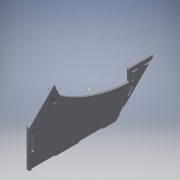
# Autodesk Inventor part: lateral
Saved by Autodesk Inventor 2016 (Build 200138000, 138)
## iProperties
Created: 2017-06-05
Part Number: lateral
Material: Genérico
Document SubType Name: Modeling
Designer: Fabio
Density: 1 g/cm^3
Appearance: Padrão
Author: Fabio
Autodesk Inventor part; units mm, degrees
ref_plane "YZ Plane" through (0, 0, 0) normal (1, 0, 0) x (0, 1, 0)
ref_plane "XZ Plane" through (0, 0, 0) normal (0, 1, 0) x (-1, 0, 0)
ref_plane "XY Plane" through (0, 0, 0) normal (0, 0, 1) x (1, 0, 0)
sketch "Esboço1" plane through (0, 0, 0) normal (1, 0, 0) x (0, 1, 0)
  line L0 (-220, 137.5) -> (220, 137.5)
  line L1 (220, 137.5) -> (220, -137.5)
  line L2 (220, -137.5) -> (-220, -137.5)
  line L3 (-220, -137.5) -> (-220, 137.5)
  point P0 (0, 0)
  point P1 (220, 0)
  point P2 (0, -137.5)
  dimension "d0" = 440
  dimension "d1" = 275
  constraints: 8 end point, 2 midpoint, 2 parallel, 1 horizontal, 1 horizontal alignment, 1 perpendicular, 1 vertical alignment
  measures "d0" distance between parallel lines of L3 L1
  measures "d1" distance between parallel lines of L0 L2
extrude "Extrusão1" add sketch "Esboço1" along normal blind 8
sketch "Esboço2" plane through (8, 0, 0) normal (1, 0, 0) x (0, 0, -1)
  line L0 (124.1566, 220.0243) -> (0, 220)
  line L1 (137.5, 220) -> (-137.5, 220) projected
  line L2 (0, 135) -> (42.099, 135)
  line L3 (0, 135) -> (0, 220)
  line L4 (-137.5, -220) -> (137.5, -220) projected
  line L5 (137.5, 220) -> (137.5, -220)
  line L6 (137.5, -220) -> (-137.5, -220)
  line L7 (-137.5, -220) -> (-137.5, -140)
  line L8 (-137.5, 220) -> (-137.5, -220) projected
  arc A0 (-137.5, -140) -> (-37.6456, -108.3893) centre (-153.3983, 83.74) ccw
  arc A1 (-37.6456, -108.3893) -> (42.099, 135) centre (-427.017, 153.9438) ccw
  line L9 (137.5, -220) -> (137.5, 220) projected
  line L10 (137.5, -120) -> (-12.5, -120)
  line L11 (-12.5, -120) -> (-127.5, -163)
  line L12 (-127.5, -163) -> (-127.5, -210)
  line L13 (-127.5, -210) -> (137.5, -210)
  line L14 (10, 145) -> (50.5, 145)
  line L15 (50.5, 145) -> (137.5, 98)
  line L16 (137.5, 98) -> (137.5, 210)
  line L17 (10, 210) -> (10, 145)
  line L18 (10, 210) -> (137.5, 210)
  line L19 (137.5, 98) -> (137.5, 210)
  point P0 (0, 0)
  dimension "d8" = 137.5
  dimension "d9" = 275
  dimension "d10" = 80
  dimension "d11" = 85
  dimension "d12" = 10
  dimension "d13" = 10
  dimension "d14" = 10
  dimension "d15" = 65
  dimension "d16" = 150
  dimension "d17" = 10
  dimension "d18" = 10
  dimension "d19" = 90
  dimension "d20" = 115
  dimension "d21" = 47
  dimension "d22" = 112
  dimension "d23" = 87
  dimension "d24" = 420
  dimension "d25" = 40.5
  constraints: 32 end point, 5 point on line, 4 perpendicular, 4 point on circle, 2 centre point, 2 collinear, 2 horizontal, 2 vertical, 1 midpoint, 1 parallel
  measures "d8" distance between parallel lines of L5 L3
  measures "d9" distance between parallel lines of L5 L7
  measures "d10" distance of L4.start L7.end
  measures "d11" distance between parallel lines of L1 L2
  measures "d12" distance between parallel lines of L2 L14
  measures "d13" distance between parallel lines of L1 L18
  measures "d14" distance between parallel lines of L3 L17
  measures "d15" distance between parallel lines of L18 L14
  measures "d16" distance of L10.start L10.end
  measures "d17" distance between parallel lines of L8 L12
  measures "d18" distance between parallel lines of L4 L13
  measures "d19" distance between parallel lines of L13 L10
  measures "d20" horizontal distance of L10.end L11.end
  measures "d21" distance from line of L11.end L13
  measures "d22" distance of L16.end L15.end
  measures "d23" horizontal distance of L14.end L15.end
  measures "d24" distance between parallel lines of L13 L18
  measures "d25" distance of L14.start L14.end
extrude "Extrusão2" cut sketch "Esboço2" against normal blind 10 contours L3 L2 A1 A0 L8 L1
fillet "Arredondamento1" radius 4 7 edges at (4, 135, 0) (4, 135, -42.099) (4, 220, 0) (4, 220, -137.5) (4, -140, 137.5) (4, -220, 137.5) (4, -220, -137.5)
fillet "Arredondamento2" radius 40 1 edges at (4, -108.3893, 37.6456)
sketch "Esboço3" plane through (0, 0, 0) normal (-1, 0, 0) x (0, 0, 1)
  point P0 (0, 0)
sketch "Esboço4" plane through (0, 0, 0) normal (-1, 0, 0) x (0, 0, 1)
  point P0 (0, 0)
sketch "Esboço5" plane through (8, 0, 0) normal (1, 0, 0) x (0, 0, -1)
  line L0 (-123.5, -210) -> (-119.5, -210)
  line L1 (-119.5, -210) -> (-119.5, -194)
  line L2 (-119.5, -194) -> (-123.5, -194)
  line L3 (-123.5, -194) -> (-123.5, -210)
  line L4 (-137.5, -143.6953) -> (-137.5, -216) projected
  line L5 (-133.5, -220) -> (133.5, -220) projected
  circle A0 centre (-123.5, -194) radius 1
  circle A1 centre (-119.5, -194) radius 1
  circle A2 centre (-123.5, -210) radius 1
  circle A3 centre (-119.5, -210) radius 1
  line L6 (-123.5, -178) -> (-119.5, -178)
  line L7 (-119.5, -178) -> (-119.5, -162)
  line L8 (-119.5, -162) -> (-123.5, -162)
  line L9 (-123.5, -162) -> (-123.5, -178)
  circle A4 centre (-119.5, -178) radius 1
  circle A5 centre (-123.9206, -178) radius 1
  circle A6 centre (-123.5, -162) radius 1
  circle A7 centre (-119.5, -162) radius 1
  point P0 (0, 0)
  dimension "d26" = 14
  dimension "d27" = 10
  dimension "d28" = 4
  dimension "d29" = 16
  dimension "d30" = 2
  dimension "d31" = 2
  dimension "d32" = 2
  dimension "d33" = 2
  dimension "d36" = 4
  dimension "d37" = 16
  dimension "d38" = 16
  dimension "d39" = 2
  dimension "d40" = 2
  dimension "d41" = 2
  dimension "d42" = 2
  constraints: 16 end point, 8 centre point, 7 coincident, 4 parallel, 2 horizontal, 2 perpendicular, 1 point on line
  measures "d26" distance between parallel lines of L4 L3
  measures "d27" distance between parallel lines of L5 L0
  measures "d28" distance between parallel lines of L3 L1
  measures "d29" distance between parallel lines of L2 L0
  measures "d30" diameter of A0
  measures "d31" diameter of A1
  measures "d32" diameter of A2
  measures "d33" diameter of A3
  measures "d36" distance of L8.end L7.end
  measures "d37" distance between parallel lines of L8 L6
  measures "d38" distance between parallel lines of L2 L6
  measures "d39" diameter of A4
  measures "d40" diameter of A5
  measures "d41" diameter of A6
  measures "d42" diameter of A7
extrude "Extrusão3" cut sketch "Esboço5" against normal blind 10
sketch "Esboço6" plane through (0, 0, 0) normal (-1, 0, 0) x (0, 0, 1)
  line L0 (-133.5, -220) -> (133.5, -220) projected
  line L1 (137.5, -216) -> (137.5, -143.6953) projected
  line L2 (119.777, -158.218) -> (118.4964, -162.0075)
  line L3 (1.0227, -122.3095) -> (2.3033, -118.52)
  line L4 (95.7596, -154.324) -> (97.0402, -150.5345)
  line L5 (72.4086, -142.2107) -> (71.128, -146.0002)
  line L6 (49.6717, -134.5273) -> (48.3912, -138.3167)
  line L7 (48.3912, -138.3167) -> (23.7596, -129.993)
  line L8 (25.0401, -126.2035) -> (49.6717, -134.5273)
  line L9 (71.128, -146.0002) -> (95.7596, -154.324)
  line L10 (97.0402, -150.5345) -> (72.4086, -142.2107)
  line L11 (23.7596, -129.993) -> (25.0401, -126.2035)
  circle A0 centre (71.128, -146.0002) radius 1
  circle A1 centre (72.4086, -142.2107) radius 1
  circle A2 centre (95.7596, -154.324) radius 1
  circle A3 centre (97.0402, -150.5345) radius 1
  circle A4 centre (48.3912, -138.3167) radius 1
  circle A5 centre (49.6717, -134.5273) radius 1
  circle A6 centre (23.7596, -129.993) radius 1
  circle A7 centre (25.0401, -126.2035) radius 1
  point P0 (0, 0)
  dimension "d43" = 61.782
  dimension "d44" = 17.723
  dimension "d45" = 101.48
  dimension "d47" = 4
  dimension "d50" = 24
  dimension "d51" = 26
  dimension "d52" = 26
  dimension "d53" = 24
  dimension "d54" = 2
  dimension "d55" = 2
  dimension "d56" = 2
  dimension "d57" = 2
  dimension "d58" = 2
  dimension "d59" = 2
  dimension "d60" = 2
  dimension "d61" = 2
  constraints: 20 end point, 8 centre point, 8 coincident, 2 perpendicular
  measures "d43" distance from line of L0 L2.start
  measures "d44" distance from line of L1 L2.start
  measures "d45" distance from line of L0 L3.end
  measures "d47" distance of L2.start L2.end
  measures "d50" distance between parallel lines of L2 L4
  measures "d51" distance between parallel lines of L5 L4
  measures "d52" distance between parallel lines of L11 L6
  measures "d53" distance from line of L6.start L5
  measures "d54" diameter of A0
  measures "d55" diameter of A1
  measures "d56" diameter of A2
  measures "d57" diameter of A3
  measures "d58" diameter of A4
  measures "d59" diameter of A5
  measures "d60" diameter of A6
  measures "d61" diameter of A7
extrude "Extrusão4" cut sketch "Esboço6" against normal blind 10
sketch "Esboço7" plane through (0, 0, 0) normal (-1, 0, 0) x (0, 0, 1)
  line L0 (-137.5, 216) -> (-137.5, -216) projected
  line L1 (-137.5, -210) -> (-133.5, -210)
  line L2 (-133.5, -210) -> (-133.5, -126)
  line L3 (-133.5, -126) -> (-137.5, -126)
  line L4 (-137.5, -126) -> (-137.5, -210)
  line L5 (-133.5, -220) -> (133.5, -220) projected
  line L6 (-137.5, -216) -> (-137.5, 216) projected
  line L7 (-137.5, -42) -> (-133.5, -42)
  line L8 (-133.5, -42) -> (-133.5, 42)
  line L9 (-133.5, 42) -> (-137.5, 42)
  line L10 (-137.5, 42) -> (-137.5, -42)
  line L11 (-137.5, 126) -> (-133.5, 126)
  line L12 (-133.5, 126) -> (-133.5, 210)
  line L13 (-133.5, 210) -> (-137.5, 210)
  line L14 (-137.5, 210) -> (-137.5, 126)
  circle A0 centre (-133.5, 210) radius 1
  circle A1 centre (-133.5, 126) radius 1
  circle A2 centre (-133.5, 42) radius 1
  circle A3 centre (-133.5, -42) radius 1
  circle A4 centre (-133.5, -126) radius 1
  circle A5 centre (-133.5, -210) radius 1
  point P0 (0, 0)
  dimension "d62" = 4
  dimension "d63" = 84
  dimension "d64" = 10
  dimension "d65" = 4
  dimension "d66" = 84
  dimension "d67" = 84
  dimension "d68" = 84
  dimension "d69" = 84
  dimension "d70" = 2
  dimension "d71" = 2
  dimension "d72" = 2
  dimension "d73" = 2
  dimension "d74" = 2
  dimension "d75" = 2
  constraints: 24 end point, 6 centre point, 6 coincident, 6 parallel, 3 horizontal, 3 perpendicular, 3 point on line
  measures "d62" distance of L3.end L2.end
  measures "d63" distance between parallel lines of L3 L1
  measures "d64" distance between parallel lines of L5 L1
  measures "d65" distance of L9.end L8.end
  measures "d66" distance between parallel lines of L9 L7
  measures "d67" distance from line of L7.start L3
  measures "d68" distance between parallel lines of L13 L11
  measures "d69" distance between parallel lines of L9 L11
  measures "d70" diameter of A0
  measures "d71" diameter of A1
  measures "d72" diameter of A2
  measures "d73" diameter of A3
  measures "d74" diameter of A4
  measures "d75" diameter of A5
extrude "Extrusão5" cut sketch "Esboço7" against normal blind 10
sketch "Esboço8" plane through (0, 0, 0) normal (-1, 0, 0) x (0, 0, 1)
  line L0 (-97.5, 210) -> (-54, 210)
  line L1 (-54, 210) -> (-54, 206)
  line L2 (-54, 206) -> (-97.5, 206)
  line L3 (-97.5, 206) -> (-97.5, 210)
  line L4 (-4, 220) -> (-133.5, 220) projected
  line L5 (-137.5, 216) -> (-137.5, 210) projected
  circle A0 centre (-97.5, 210) radius 1
  circle A1 centre (-97.5, 206) radius 1
  circle A2 centre (-54, 210) radius 1
  circle A3 centre (-54, 206) radius 1
  point P0 (0, 0)
  dimension "d78" = 10
  dimension "d79" = 4
  dimension "d80" = 40
  dimension "d81" = 43.5
  dimension "d82" = 2
  dimension "d83" = 2
  dimension "d84" = 2
  dimension "d85" = 2
  constraints: 8 end point, 4 centre point, 4 coincident, 2 parallel, 1 horizontal, 1 perpendicular
  measures "d78" distance between parallel lines of L4 L0
  measures "d79" distance between parallel lines of L2 L0
  measures "d80" distance between parallel lines of L5 L3
  measures "d81" distance between parallel lines of L1 L3
  measures "d82" diameter of A0
  measures "d83" diameter of A1
  measures "d84" diameter of A2
  measures "d85" diameter of A3
extrude "Extrusão6" cut sketch "Esboço8" against normal blind 10
sketch "Esboço9" plane through (0, 0, 0) normal (-1, 0, 0) x (0, 0, 1)
  line L0 (-14, 210) -> (-18, 210)
  line L1 (-18, 210) -> (-18, 190)
  line L2 (-18, 190) -> (-14, 190)
  line L3 (-14, 190) -> (-14, 210)
  line L4 (-4, 220) -> (-133.5, 220) projected
  line L5 (0, 139) -> (0, 216) projected
  line L6 (-18, 145) -> (-14, 145)
  line L7 (-14, 145) -> (-14, 165)
  line L8 (-14, 165) -> (-18, 165)
  line L9 (-18, 165) -> (-18, 145)
  circle A0 centre (-18, 210) radius 1
  circle A1 centre (-14, 210) radius 1
  circle A2 centre (-18, 190) radius 1
  circle A3 centre (-14, 190) radius 1
  circle A4 centre (-18, 165) radius 1
  circle A5 centre (-14, 165) radius 1
  circle A6 centre (-18, 145) radius 1
  circle A7 centre (-14, 145) radius 1
  point P0 (0, 0)
  dimension "d88" = 4
  dimension "d89" = 10
  dimension "d90" = 14
  dimension "d91" = 20
  dimension "d92" = 20
  dimension "d93" = 25
  dimension "d94" = 2
  dimension "d95" = 2
  dimension "d96" = 2
  dimension "d97" = 2
  dimension "d98" = 2
  dimension "d99" = 2
  dimension "d100" = 2
  dimension "d103" = 4
  dimension "d104" = 14
  constraints: 16 end point, 8 centre point, 8 coincident, 4 parallel, 2 horizontal, 2 perpendicular
  measures "d88" distance of L2.end L1.end
  measures "d89" distance between parallel lines of L4 L0
  measures "d90" distance between parallel lines of L5 L3
  measures "d91" distance between parallel lines of L0 L2
  measures "d92" distance between parallel lines of L6 L8
  measures "d93" distance between parallel lines of L2 L8
  measures "d94" diameter of A0
  measures "d95" diameter of A1
  measures "d96" diameter of A2
  measures "d97" diameter of A4
  measures "d98" diameter of A5
  measures "d99" diameter of A6
  measures "d100" diameter of A7
  measures "d103" distance between parallel lines of L7 L9
  measures "d104" distance between parallel lines of L5 L7
extrude "Extrusão7" cut sketch "Esboço9" against normal blind 10
sketch "Esboço10" plane through (0, 0, 0) normal (-1, 0, 0) x (0, 0, 1)
  line L0 (-28, 149) -> (-44.5, 149)
  line L1 (-44.5, 149) -> (-44.5, 145)
  line L2 (-44.5, 145) -> (-28, 145)
  line L3 (-28, 145) -> (-28, 149)
  line L4 (-37.9156, 135) -> (-4, 135) projected
  line L5 (0, 139) -> (0, 216) projected
  circle A0 centre (-44.5, 149) radius 1
  circle A1 centre (-44.5, 145) radius 1
  circle A2 centre (-28, 149) radius 1
  circle A3 centre (-28, 145) radius 1
  point P0 (0, 0)
  dimension "d105" = 16.5
  dimension "d106" = 4
  dimension "d107" = 10
  dimension "d108" = 28
  dimension "d109" = 2
  dimension "d110" = 2
  dimension "d111" = 2
  dimension "d112" = 2
  constraints: 8 end point, 4 centre point, 4 coincident, 2 parallel, 1 horizontal, 1 perpendicular
  measures "d105" distance of L2.end L1.end
  measures "d106" distance of L1.end L0.end
  measures "d107" distance between parallel lines of L4 L2
  measures "d108" distance between parallel lines of L5 L3
  measures "d109" diameter of A0
  measures "d110" diameter of A1
  measures "d111" diameter of A2
  measures "d112" diameter of A3
extrude "Extrusão8" cut sketch "Esboço10" against normal blind 10
sketch "Esboço11" plane through (0, 0, 0) normal (-1, 0, 0) x (0, 0, 1)
  line L0 (0, 139) -> (0, 216) projected
  line L1 (-4, 220) -> (-133.5, 220) projected
  line L2 (-137.5, 126) -> (-137.5, 42) projected
  line L3 (-82.61, 132.568) -> (-80.292, 129.308)
  line L4 (-80.292, 129.308) -> (-59.9175, 143.7952)
  line L5 (-59.9175, 143.7952) -> (-62.2355, 147.0552)
  line L6 (-62.2355, 147.0552) -> (-82.61, 132.568)
  line L7 (-103.7995, 117.5013) -> (-101.4815, 114.2413)
  line L8 (-101.4815, 114.2413) -> (-121.8561, 99.7542)
  line L9 (-121.8561, 99.7542) -> (-124.1741, 103.0142)
  line L10 (-124.1741, 103.0142) -> (-103.7995, 117.5013)
  circle A0 centre (-82.61, 132.568) radius 1
  circle A1 centre (-80.292, 129.308) radius 1
  circle A2 centre (-59.9175, 143.7952) radius 1
  circle A3 centre (-62.2355, 147.0552) radius 1
  circle A4 centre (-103.7995, 117.5013) radius 1
  circle A5 centre (-101.4815, 114.2413) radius 1
  circle A6 centre (-124.1741, 103.0142) radius 1
  circle A7 centre (-121.8561, 99.7542) radius 1
  point P0 (0, 0)
  dimension "d115" = 82.61
  dimension "d116" = 87.432
  dimension "d117" = 90.692
  dimension "d118" = 57.208
  dimension "d119" = 25
  dimension "d120" = 26
  dimension "d121" = 25
  dimension "d122" = 2
  dimension "d123" = 2
  dimension "d124" = 2
  dimension "d125" = 2
  dimension "d126" = 2
  dimension "d127" = 2
  dimension "d128" = 2
  dimension "d129" = 2
  constraints: 16 end point, 8 centre point, 8 coincident, 5 perpendicular
  measures "d115" distance from line of L0 L3.start
  measures "d116" distance from line of L1 L3.start
  measures "d117" distance from line of L1 L3.end
  measures "d118" distance from line of L2 L3.end
  measures "d119" distance of L3.end L4.end
  measures "d120" distance of L3.start L7.start
  measures "d121" distance of L7.end L8.end
  measures "d122" diameter of A0
  measures "d123" diameter of A1
  measures "d124" diameter of A2
  measures "d125" diameter of A3
  measures "d126" diameter of A4
  measures "d127" diameter of A5
  measures "d128" diameter of A6
  measures "d129" diameter of A7
extrude "Extrusão9" cut sketch "Esboço11" against normal blind 10
sketch "Esboço12" plane through (0, 0, 0) normal (-1, 0, 0) x (0, 0, 1)
  line L0 (70.5, -210) -> (19.5, -210)
  line L1 (19.5, -210) -> (19.5, -202)
  line L2 (19.5, -202) -> (70.5, -202)
  line L3 (70.5, -202) -> (70.5, -210)
  line L4 (137.5, -216) -> (137.5, -143.6953) projected
  line L5 (-133.5, -220) -> (133.5, -220) projected
  line L6 (-33.5, -202) -> (-84.5, -202)
  line L7 (-84.5, -202) -> (-84.5, -210)
  line L8 (-84.5, -210) -> (-33.5, -210)
  line L9 (-33.5, -210) -> (-33.5, -202)
  circle A0 centre (-84.5, -202) radius 1
  circle A1 centre (-84.5, -210) radius 1
  circle A2 centre (-33.5, -210) radius 1
  circle A3 centre (-33.5, -202) radius 1
  circle A4 centre (19.5, -202) radius 1
  circle A5 centre (19.5, -210) radius 1
  circle A6 centre (70.5, -210) radius 1
  circle A7 centre (70.5, -202) radius 1
  point P0 (0, 0)
  dimension "d132" = 8
  dimension "d133" = 67
  dimension "d134" = 10
  dimension "d135" = 51
  dimension "d136" = 51
  dimension "d137" = 53
  dimension "d138" = 2
  dimension "d139" = 2
  dimension "d140" = 2
  dimension "d141" = 2
  dimension "d142" = 2
  dimension "d143" = 2
  constraints: 16 end point, 8 centre point, 8 coincident, 4 parallel, 2 horizontal, 2 perpendicular
  measures "d132" distance of L0.end L1.end
  measures "d133" distance between parallel lines of L4 L3
  measures "d134" distance between parallel lines of L5 L0
  measures "d135" distance between parallel lines of L1 L3
  measures "d136" distance between parallel lines of L7 L9
  measures "d137" distance between parallel lines of L1 L9
  measures "d138" diameter of A0
  measures "d139" diameter of A1
  measures "d140" diameter of A2
  measures "d141" diameter of A3
  measures "d142" diameter of A4
  measures "d143" diameter of A5
extrude "Extrusão10" cut sketch "Esboço12" against normal blind 10
